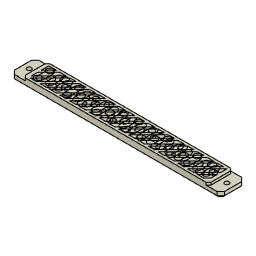
Front Panel - Master (Autodesk Fusion 360 design; units mm, degrees)
Autodesk Fusion 360 part; units mm, degrees
ref_plane "WorkPlane1" through (0, -117.8, 0) normal (0, 1, 0) x (0, 0, 1)
ref_plane "WorkPlane2" through (0, -123, 0) normal (0, 1, 0) x (0, 0, 1)
sketch "Master Sketch" plane through (0, -123, 0) normal (0, 1, 0) x (1, 0, 0)
  line L0 (-88.4862, 0.0071) -> (88.5, 0.0071) construction
  line L1 (88.5, 0.0071) -> (88.5, -28.9292)
  line L2 (88.5, -28.9292) -> (87.9405, -29.5447) construction
  line L3 (-88.4655, 0) -> (-88.4655, -26.8517) construction
  line L4 (-88.4862, -26.8517) -> (89.2, -26.8517) construction
  line L5 (89.2, -26.8517) -> (89.2, 0) construction
  line L6 (88.5, -26.8517) -> (88.5, 0.0071)
  line L7 (-88.4862, -26.8517) -> (88.5, -26.8517)
  line L8 (88.5, 0.0071) -> (-88.4862, 0.0071)
  line L9 (-88.4862, -26.8517) -> (-88.4862, 0.0071)
  line L10 (85.5, -21.8517) -> (85.5, -7.8517)
  line L11 (-82.4864, -24.8517) -> (82.5, -24.8517)
  line L12 (82.5, -4.8517) -> (-82.4864, -4.8517)
  line L13 (-88.4655, -4.8517) -> (-88.5, -4.8517)
  line L14 (-85.4864, -21.8517) -> (-85.4864, -7.8517)
  line L15 (-85.4864, 0.0071) -> (-85.4864, 0.0039)
  line L16 (-75.4864, -24.8517) -> (-75.4864, -4.8517)
  line L17 (75.5, -24.8517) -> (75.5, -4.8517)
  line L18 (-75.4864, -4.8517) -> (-80.4972, -4.8517)
  line L19 (-85.4864, -24.8517) -> (-75.4864, -24.8517) construction
  line L20 (-80.4864, -24.8517) -> (-80.4972, -4.8517) construction
  line L21 (0.0068, -24.8517) -> (0.0068, -4.8517) construction
  arc A0 (-82.4864, -4.8517) -> (-85.4864, -7.8517) centre (-82.4864, -7.8517) ccw construction
  arc A1 (-85.4864, -21.8517) -> (-82.4864, -24.8517) centre (-82.4864, -21.8517) ccw construction
  arc A2 (85.5, -7.8517) -> (82.5, -4.8517) centre (82.5, -7.8517) ccw construction
  arc A3 (82.5, -24.8517) -> (85.5, -21.8517) centre (82.5, -21.8517) ccw construction
  circle A4 centre (-80.4836, -14.7936) radius 1.8
  circle A5 centre (80.4971, -14.7936) radius 1.8
  line L22 (-85.4864, -21.8517) -> (-82.4864, -24.8517)
  line L23 (-85.4864, -7.8517) -> (-82.4864, -4.8517)
  line L24 (85.5, -7.8517) -> (82.5, -4.8517)
  line L25 (85.5, -21.8517) -> (82.4977, -24.8517)
  point P0 (85.5, -4.8517)
  point P1 (85.5, -24.8517)
  dimension "d919" = 2
  dimension "d922" = 20
  dimension "d925" = 10
  dimension "d926" = 10
  dimension "d928" = 3
  dimension "d929" = 3
  dimension "d930" = 3
  dimension "d931" = 3
  dimension "d932" = 3.6
  constraint coincident L4 L6.start
  constraint coincident L1 L6.start
  constraint coincident L0.end L1.start
  constraint coincident L4.start L7.start
  constraint coincident L0.start L8.end
  constraint parallel L7 L11
  constraint parallel L9 L14
  constraint parallel L8 L12
  constraint coincident L3 L13.start
  constraint collinear L12 L13
  constraint coincident L0 L15.start
  constraint collinear L14 L15
  constraint parallel L6 L10
  constraint parallel L10 L17
  constraint coincident L11 L17.start
  constraint coincident L12 L17.end
  constraint parallel L14 L16
  constraint perpendicular L14 L18
  constraint perpendicular L16 L19
  constraint midpoint L19 L20.start
  constraint coincident L12 L21.end
  constraint tangent L12 A0
  constraint tangent L14 A0
  constraint coincident L11 L21.start
  constraint coincident L19.start L14
  constraint coincident L11 L19.start
  constraint tangent L14 A1
  constraint tangent L11 A1
  constraint coincident L12 P0
  constraint coincident L10 P0
  constraint tangent L12 A2
  constraint tangent L10 A2
  constraint coincident L11 P1
  constraint coincident L10 P1
  constraint tangent L11 A3
  constraint tangent L10 A3
  constraint symmetric L21 A4 A5
  constraint coincident L12 L16.end
  constraint coincident L11 L16.start
  constraint vertical L16
  constraint horizontal L12
  constraint vertical L10
  constraint symmetric L21 L12.end L12.start
  constraint symmetric L21 L14.end L10.end
  constraint symmetric L21 L14.start L10.start
  constraint coincident L11 L25.end
  constraint coincident L10 A3.end
  constraint coincident L10 A2.start
  measures "d919" distance of L7 L11
  measures "d922" distance of P0 P1
  measures "d925" distance of L10 L17
  measures "d926" distance of L14 L16
  measures "d928" radius of A0
  measures "d929" radius of A1
  measures "d930" radius of A2
  measures "d931" radius of A3
  measures "d932" diameter of A4
extrude "Extrude1" add sketch "Master Sketch" along normal blind 4 contours L11 L12 L16 L17 makes body 1
extrude "Extrude2" add sketch "Master Sketch" along normal blind 2 contours L10 L11 L12 L17 L24 L25 | L11 L12 L14 L16 L18 L22 L23 bodies 1
chamfer "Chamfer1" distance 2 angle 45 4 edges at (-75.4864, -120, 24.8517) (-75.4864, -120, 4.8517) (75.5, -120, 4.8517) (75.5, -120, 24.8517) on bodies 1
move_body "Move1" bodies 1 to x (1, 0, 0) y (0, 0, 1) z (0, -1, 0) at (0, -118.1483, 127.8517)
extrude "Extrude3" add 3 faces at (-25.1576, -129.6667, 4.8517) (-79.352, -140.2322, 4.8517) (79.3648, -140.2322, 4.8517) along direction (0, 0, -1) blind 3 on bodies 1 bodies 1
chamfer "Chamfer2" distance 2 angle 45 8 edges at (85.5, -133, 1.8517) (83.9988, -141.5, 1.8517) (0.0056, -143, 1.8517) (-83.9864, -141.5, 1.8517) (-85.4864, -133, 1.8517) (-83.9864, -124.5, 1.8517) (0.0068, -123, 1.8517) (84, -124.5, 1.8517) on bodies 1
copy_body "Body->Comp1" bodies 1 removing the originals makes body 2 in component "Master"
sketch "Outline" plane through (0, -117.8, 0) normal (0, 1, 0) x (1, 0, 0) in component "Master"
  line L0 (-88.4655, -26.8517) -> (89.2, -26.8517)
  line L1 (89.2, -26.8517) -> (89.2, 0)
  line L2 (89.2, 0) -> (-88.4655, 0)
  line L3 (-88.4655, 0) -> (-88.4655, -26.8517)
sketch "USB A Panel Mount" plane through (0.0068, -133, 8.8517) normal (0, 0, 1) x (-1, 0, 0) in component "USB Sketches"
  line L0 (-73.4932, 10) -> (-75.4932, 8)
  line L1 (-75.4932, 8) -> (-75.4932, -8)
  line L2 (-75.4932, -8) -> (-73.4932, -10)
  line L3 (-73.4932, -10) -> (73.4932, -10)
  line L4 (73.4932, -10) -> (75.4932, -8)
  line L5 (75.4932, -8) -> (75.4932, 8)
  line L6 (75.4932, 8) -> (73.4932, 10)
  line L7 (73.4932, 10) -> (-73.4932, 10)
  line L8 (72.4932, 7.5) -> (33.4932, 7.5)
  line L9 (33.4932, 7.5) -> (33.4932, -7.5)
  line L10 (33.4932, -7.5) -> (72.4932, -7.5)
  line L11 (72.4932, -7.5) -> (72.4932, 7.5)
  line L12 (45.7432, -6) -> (60.2432, -6)
  line L13 (60.2432, -6) -> (60.2432, 6)
  line L14 (45.7432, 6) -> (45.7432, -6)
  line L15 (60.2432, 6) -> (45.7432, 6)
  circle A0 centre (68.2432, 0) radius 1.8
  circle A1 centre (37.7432, 0) radius 1.8
sketch "USB C Panel Mount" plane through (0.0068, -133, 8.8517) normal (0, 0, 1) x (-1, 0, 0) in component "USB Sketches"
  line L0 (-73.4932, 10) -> (-75.4932, 8)
  line L1 (-75.4932, 8) -> (-75.4932, -8)
  line L2 (-75.4932, -8) -> (-73.4932, -10)
  line L3 (-73.4932, -10) -> (73.4932, -10)
  line L4 (73.4932, -10) -> (75.4932, -8)
  line L5 (75.4932, -8) -> (75.4932, 8)
  line L6 (75.4932, 8) -> (73.4932, 10)
  line L7 (73.4932, 10) -> (-73.4932, 10)
  line L8 (72.4932, 6) -> (47.4932, 6)
  line L9 (47.4932, 6) -> (47.4932, -6)
  line L10 (47.4932, -6) -> (72.4932, -6)
  line L11 (72.4932, -6) -> (72.4932, 6)
  arc A0 (63.4932, -2.5) -> (64.4932, -1.5) centre (63.4932, -1.5) ccw
  line L12 (64.4932, 0) -> (64.4932, -1.5)
  line L13 (59.9932, -2.5) -> (63.4932, -2.5)
  arc A1 (55.4932, -1.5) -> (56.4932, -2.5) centre (56.4932, -1.5) ccw
  line L14 (55.4932, 0) -> (55.4932, -1.5)
  line L15 (59.9932, -2.5) -> (56.4932, -2.5)
  arc A2 (56.4932, 2.5) -> (55.4932, 1.5) centre (56.4932, 1.5) ccw
  line L16 (55.4932, 0) -> (55.4932, 1.5)
  line L17 (59.9932, 2.5) -> (56.4932, 2.5)
  circle A3 centre (51.6182, 0) radius 1.75
  circle A4 centre (68.3682, 0) radius 1.75
  arc A5 (64.4932, 1.5) -> (63.4932, 2.5) centre (63.4932, 1.5) ccw
  line L18 (59.9932, 2.5) -> (63.4932, 2.5)
  line L19 (64.4932, 0) -> (64.4932, 1.5)
sketch "Micro SD Slot" plane through (0, 0, 8.8517) normal (0, 0, 1) x (-1, 0, 0) in component "Master"
  line L0 (-73.5, 143) -> (-75.5, 141)
  line L1 (-75.5, 141) -> (-75.5, 125)
  line L2 (-75.5, 125) -> (-73.5, 123)
  line L3 (-73.5, 123) -> (73.4864, 123)
  line L4 (73.4864, 123) -> (75.4864, 125)
  line L5 (75.4864, 125) -> (75.4864, 141)
  line L6 (75.4864, 141) -> (73.4864, 143)
  line L7 (73.4864, 143) -> (-73.5, 143)
  line L8 (26.05, 129.6) -> (2.25, 129.6)
  line L9 (2.25, 129.6) -> (2.25, 136.4)
  line L10 (2.25, 136.4) -> (26.05, 136.4)
  line L11 (26.05, 136.4) -> (26.05, 129.6)
  line L12 (14.15, 132.9821) -> (28.75, 132.9821) construction
  line L13 (14.15, 132.9821) -> (14.15, 136.4) construction
  circle A0 centre (28.75, 132.9821) radius 1.8
  circle A1 centre (-0.45, 132.9821) radius 1.8
  line L14 (33.4864, 140.5) -> (33.4864, 125.5)
  line L15 (33.4864, 125.5) -> (-5.1864, 125.5)
  line L16 (-5.1864, 125.5) -> (-5.1864, 140.4642)
  line L17 (-5.1864, 140.4642) -> (33.4864, 140.4642)
  line L18 (33.4864, 140.4642) -> (33.4864, 125.5)
  line L19 (33.4864, 125.5) -> (-5.1864, 140.4642) construction
  line L20 (-5.1864, 125.5) -> (33.4864, 140.4642) construction
  line L21 (32.65, 129.5821) -> (-4.35, 129.5821)
  line L22 (-4.35, 129.5821) -> (-4.35, 136.3821)
  line L23 (-4.35, 136.3821) -> (32.65, 136.3821)
  line L24 (32.65, 136.3821) -> (32.65, 129.5821)
  line L25 (32.65, 129.5821) -> (-4.35, 136.3821) construction
  line L26 (-4.35, 129.5821) -> (32.65, 136.3821) construction
  point P0 (14.15, 132.9821)
  point P1 (14.15, 132.9821)
  point P2 (14.15, 132.9821)
  point P3 (14.15, 132.9821)
  dimension "d11" = 23.8
  dimension "d12" = 6.8
  dimension "d13" = 14.6
  dimension "d14" = 3.6
  dimension "d48" = 37
  dimension "d49" = 6.8
  constraint horizontal L8
  constraint perpendicular L8 L9
  constraint parallel L8 L10
  constraint parallel L9 L11
  constraint coincident P3 P2
  constraint perpendicular L11 L12
  constraint midpoint L10 L13.end
  constraint perpendicular L10 L13
  constraint coincident L12.end A0.centre
  constraint symmetric L13 A0 A1
  constraint horizontal L15
  constraint perpendicular L15 L16
  constraint parallel L15 L17
  constraint parallel L16 L18
  constraint coincident L19 P3
  constraint coincident L20 P3
  constraint coincident L14.end L15.start
  constraint horizontal L21
  constraint perpendicular L21 L22
  constraint parallel L21 L23
  constraint parallel L22 L24
  constraint coincident L25 P3
  constraint coincident L26 P3
  measures "d11" distance of L9.end L10.end
  measures "d12" distance of L8.end L9.end
  measures "d13" distance of P3 L12.end
  measures "d14" diameter of A0
  measures "d48" distance of L22.end L23.end
  measures "d49" distance of L21.end L22.end
sketch "Vent Sections" plane through (0, 0, 8.8517) normal (0, 0, 1) x (-1, 0, 0) in component "Vent Sketches"
  line L0 (-73.5, 143) -> (-75.5, 141)
  line L1 (-75.5, 141) -> (-75.5, 125)
  line L2 (-75.5, 125) -> (-73.5, 123)
  line L3 (-73.5, 123) -> (73.4864, 123)
  line L4 (73.4864, 123) -> (75.4864, 125)
  line L5 (75.4864, 125) -> (75.4864, 141)
  line L6 (75.4864, 141) -> (73.4864, 143)
  line L7 (73.4864, 143) -> (-73.5, 143)
  line L8 (33.4864, 140.4642) -> (33.4864, 125.5) construction
  line L9 (-5.1864, 125.5) -> (-5.1864, 140.4642) construction
  line L10 (-72.5, 141) -> (-72.5, 125)
  line L11 (72.4864, 125) -> (72.4864, 141)
  line L12 (72.4864, 141) -> (-72.5, 141)
  line L13 (-72.5, 125) -> (72.4864, 125)
  line L14 (-5.1864, 141) -> (-5.1864, 125)
  line L15 (33.4864, 141) -> (33.4864, 125)
  dimension "d15" = -3
  dimension "d17" = -3
  constraint perpendicular L10 L12
  constraint perpendicular L11 L13
  constraint coincident L12 L14.start
  constraint coincident L13 L14.end
  constraint perpendicular L13 L14
  constraint collinear L9 L14
  constraint coincident L12 L15.start
  constraint coincident L13 L15.end
  constraint perpendicular L13 L15
  constraint collinear L8 L15
sketch "Slots" plane through (0, 0, 8.8517) normal (0, 0, 1) x (-1, 0, 0) in component "Vent Sketches"
  line L0 (-73.5, 143) -> (-75.5, 141)
  line L1 (-75.5, 141) -> (-75.5, 125)
  line L2 (-75.5, 125) -> (-73.5, 123)
  line L3 (-73.5, 123) -> (73.4864, 123)
  line L4 (73.4864, 123) -> (75.4864, 125)
  line L5 (75.4864, 125) -> (75.4864, 141)
  line L6 (75.4864, 141) -> (73.4864, 143)
  line L7 (73.4864, 143) -> (-73.5, 143)
  line L8 (72.4864, 141) -> (-72.5, 141)
  line L9 (-72.5, 141) -> (-72.5, 125)
  line L10 (-72.5, 125) -> (72.4864, 125)
  line L11 (72.4864, 125) -> (72.4864, 141)
  line L12 (-5.1864, 141) -> (-5.1864, 125)
  line L13 (33.4864, 141) -> (33.4864, 125)
  line L14 (-0.0068, 141) -> (-0.0068, 125) construction
  line L15 (2.4932, 129) -> (2.4932, 137)
  arc A0 (2.4932, 137) -> (-2.5068, 137) centre (-0.0068, 137) ccw
  line L16 (-2.5068, 137) -> (-2.5068, 129)
  arc A1 (-2.5068, 129) -> (2.4932, 129) centre (-0.0068, 129) ccw
  line L17 (-0.0068, 129) -> (-0.0068, 137) construction
  line L18 (-70.0068, 137) -> (-70.0068, 129)
  arc A2 (-70.0068, 129) -> (-65.0068, 129) centre (-67.5068, 129) ccw
  line L19 (-65.0068, 129) -> (-65.0068, 137)
  arc A3 (-65.0068, 137) -> (-70.0068, 137) centre (-67.5068, 137) ccw
  line L20 (-62.5068, 137) -> (-62.5068, 129)
  arc A4 (-62.5068, 129) -> (-57.5068, 129) centre (-60.0068, 129) ccw
  line L21 (-57.5068, 129) -> (-57.5068, 137)
  arc A5 (-57.5068, 137) -> (-62.5068, 137) centre (-60.0068, 137) ccw
  line L22 (-55.0068, 137) -> (-55.0068, 129)
  arc A6 (-55.0068, 129) -> (-50.0068, 129) centre (-52.5068, 129) ccw
  line L23 (-50.0068, 129) -> (-50.0068, 137)
  arc A7 (-50.0068, 137) -> (-55.0068, 137) centre (-52.5068, 137) ccw
  line L24 (-47.5068, 137) -> (-47.5068, 129)
  arc A8 (-47.5068, 129) -> (-42.5068, 129) centre (-45.0068, 129) ccw
  line L25 (-42.5068, 129) -> (-42.5068, 137)
  arc A9 (-42.5068, 137) -> (-47.5068, 137) centre (-45.0068, 137) ccw
  line L26 (-40.0068, 137) -> (-40.0068, 129)
  arc A10 (-40.0068, 129) -> (-35.0068, 129) centre (-37.5068, 129) ccw
  line L27 (-35.0068, 129) -> (-35.0068, 137)
  arc A11 (-35.0068, 137) -> (-40.0068, 137) centre (-37.5068, 137) ccw
  line L28 (-32.5068, 137) -> (-32.5068, 129)
  arc A12 (-32.5068, 129) -> (-27.5068, 129) centre (-30.0068, 129) ccw
  line L29 (-27.5068, 129) -> (-27.5068, 137)
  arc A13 (-27.5068, 137) -> (-32.5068, 137) centre (-30.0068, 137) ccw
  line L30 (-25.0068, 137) -> (-25.0068, 129)
  arc A14 (-25.0068, 129) -> (-20.0068, 129) centre (-22.5068, 129) ccw
  line L31 (-20.0068, 129) -> (-20.0068, 137)
  arc A15 (-20.0068, 137) -> (-25.0068, 137) centre (-22.5068, 137) ccw
  line L32 (-17.5068, 137) -> (-17.5068, 129)
  arc A16 (-17.5068, 129) -> (-12.5068, 129) centre (-15.0068, 129) ccw
  line L33 (-12.5068, 129) -> (-12.5068, 137)
  arc A17 (-12.5068, 137) -> (-17.5068, 137) centre (-15.0068, 137) ccw
  line L34 (-10.0068, 137) -> (-10.0068, 129)
  arc A18 (-10.0068, 129) -> (-5.0068, 129) centre (-7.5068, 129) ccw
  line L35 (-5.0068, 129) -> (-5.0068, 137)
  arc A19 (-5.0068, 137) -> (-10.0068, 137) centre (-7.5068, 137) ccw
  line L36 (4.9932, 137) -> (4.9932, 129)
  arc A20 (4.9932, 129) -> (9.9932, 129) centre (7.4932, 129) ccw
  line L37 (9.9932, 129) -> (9.9932, 137)
  arc A21 (9.9932, 137) -> (4.9932, 137) centre (7.4932, 137) ccw
  line L38 (12.4932, 137) -> (12.4932, 129)
  arc A22 (12.4932, 129) -> (17.4932, 129) centre (14.9932, 129) ccw
  line L39 (17.4932, 129) -> (17.4932, 137)
  arc A23 (17.4932, 137) -> (12.4932, 137) centre (14.9932, 137) ccw
  line L40 (19.9932, 137) -> (19.9932, 129)
  arc A24 (19.9932, 129) -> (24.9932, 129) centre (22.4932, 129) ccw
  line L41 (24.9932, 129) -> (24.9932, 137)
  arc A25 (24.9932, 137) -> (19.9932, 137) centre (22.4932, 137) ccw
  line L42 (27.4932, 137) -> (27.4932, 129)
  arc A26 (27.4932, 129) -> (32.4932, 129) centre (29.9932, 129) ccw
  line L43 (32.4932, 129) -> (32.4932, 137)
  arc A27 (32.4932, 137) -> (27.4932, 137) centre (29.9932, 137) ccw
  line L44 (34.9932, 137) -> (34.9932, 129)
  arc A28 (34.9932, 129) -> (39.9932, 129) centre (37.4932, 129) ccw
  line L45 (39.9932, 129) -> (39.9932, 137)
  arc A29 (39.9932, 137) -> (34.9932, 137) centre (37.4932, 137) ccw
  line L46 (42.4932, 137) -> (42.4932, 129)
  arc A30 (42.4932, 129) -> (47.4932, 129) centre (44.9932, 129) ccw
  line L47 (47.4932, 129) -> (47.4932, 137)
  arc A31 (47.4932, 137) -> (42.4932, 137) centre (44.9932, 137) ccw
  line L48 (49.9932, 137) -> (49.9932, 129)
  arc A32 (49.9932, 129) -> (54.9932, 129) centre (52.4932, 129) ccw
  line L49 (54.9932, 129) -> (54.9932, 137)
  arc A33 (54.9932, 137) -> (49.9932, 137) centre (52.4932, 137) ccw
  line L50 (57.4932, 137) -> (57.4932, 129)
  arc A34 (57.4932, 129) -> (62.4932, 129) centre (59.9932, 129) ccw
  line L51 (62.4932, 129) -> (62.4932, 137)
  arc A35 (62.4932, 137) -> (57.4932, 137) centre (59.9932, 137) ccw
  line L52 (64.9932, 137) -> (64.9932, 129)
  arc A36 (64.9932, 129) -> (69.9932, 129) centre (67.4932, 129) ccw
  line L53 (69.9932, 129) -> (69.9932, 137)
  arc A37 (69.9932, 137) -> (64.9932, 137) centre (67.4932, 137) ccw
  point P0 (-0.0068, 133)
  dimension "d18" = 5
  dimension "d21" = 7.5
  dimension "d22" = 0
  constraint midpoint L8 L14.start
  constraint midpoint L10 L14.end
  constraint tangent L15 A0
  constraint tangent A0 L16
  constraint parallel L15 L16
  constraint tangent L16 A1
  constraint tangent L15 A1
  constraint perpendicular L8 L17
  constraint midpoint L14 P0
  constraint midpoint L17 P0
  measures "d18" diameter of A0
sketch "Slats" plane through (0, 0, 8.8517) normal (0, 0, 1) x (-1, 0, 0) in component "Vent Sketches"
  line L0 (-73.5, 143) -> (-75.5, 141)
  line L1 (-75.5, 141) -> (-75.5, 125)
  line L2 (-75.5, 125) -> (-73.5, 123)
  line L3 (-73.5, 123) -> (73.4864, 123)
  line L4 (73.4864, 123) -> (75.4864, 125)
  line L5 (75.4864, 125) -> (75.4864, 141)
  line L6 (75.4864, 141) -> (73.4864, 143)
  line L7 (73.4864, 143) -> (-73.5, 143)
  line L8 (72.4864, 141) -> (-72.5, 141)
  line L9 (-72.5, 141) -> (-72.5, 125)
  line L10 (72.4864, 125) -> (72.4864, 141)
  line L11 (-72.5, 125) -> (72.4864, 125)
  line L12 (-5.1864, 141) -> (-5.1864, 125)
  line L13 (33.4864, 141) -> (33.4864, 125)
  line L14 (-72.5, 125) -> (-56.4903, 141)
  line L15 (-69.5, 125) -> (-53.4903, 141)
  line L16 (-61.5, 125) -> (-45.4903, 141)
  line L17 (-64.5, 125) -> (-48.4903, 141)
  line L18 (-53.5, 125) -> (-37.4903, 141)
  line L19 (-56.5, 125) -> (-40.4903, 141)
  line L20 (-45.5, 125) -> (-29.4903, 141)
  line L21 (-48.5, 125) -> (-32.4903, 141)
  line L22 (-37.5, 125) -> (-21.4903, 141)
  line L23 (-40.5, 125) -> (-24.4903, 141)
  line L24 (-29.5, 125) -> (-13.4903, 141)
  line L25 (-32.5, 125) -> (-16.4903, 141)
  line L26 (-21.5, 125) -> (-5.4903, 141)
  line L27 (-24.5, 125) -> (-8.4903, 141)
  line L28 (-13.5, 125) -> (2.5097, 141)
  line L29 (-16.5, 125) -> (-0.4903, 141)
  line L30 (-5.5, 125) -> (10.5097, 141)
  line L31 (-8.5, 125) -> (7.5097, 141)
  line L32 (2.5, 125) -> (18.5097, 141)
  line L33 (-0.5, 125) -> (15.5097, 141)
  line L34 (10.5, 125) -> (26.5097, 141)
  line L35 (7.5, 125) -> (23.5097, 141)
  line L36 (18.5, 125) -> (34.5097, 141)
  line L37 (15.5, 125) -> (31.5097, 141)
  line L38 (26.5, 125) -> (42.5097, 141)
  line L39 (23.5, 125) -> (39.5097, 141)
  line L40 (34.5, 125) -> (50.5097, 141)
  line L41 (31.5, 125) -> (47.5097, 141)
  line L42 (42.5, 125) -> (58.5097, 141)
  line L43 (39.5, 125) -> (55.5097, 141)
  line L44 (50.5, 125) -> (66.5097, 141)
  line L45 (47.5, 125) -> (63.5097, 141)
  line L46 (58.5, 125) -> (74.5097, 141)
  line L47 (55.5, 125) -> (71.5097, 141)
  line L48 (66.5, 125) -> (82.5097, 141)
  line L49 (63.5, 125) -> (79.5097, 141)
  line L50 (-72.5, 137.9921) -> (-69.4903, 141)
  line L51 (-72.5, 140.9903) -> (-72.4903, 141)
  line L52 (-72.5, 132.9951) -> (-64.4903, 141)
  line L53 (-72.5, 129.997) -> (-61.4903, 141)
  dimension "d25" = 8
  dimension "d26" = 0
  constraint coincident L9.end L11.start
  constraint coincident L8 L14.end
  constraint coincident L8 L15.end
  constraint coincident L11 L15.start
  constraint parallel L14 L15
  constraint coincident L9 L50.start
  constraint coincident L9 L51.start
  constraint coincident L9 L52.start
  constraint coincident L9 L53.start
sketch "Hexagons" plane through (0, 0, 8.8517) normal (0, 0, 1) x (-1, 0, 0) in component "Vent Sketches"
  line L0 (-73.5, 143) -> (-75.5, 141)
  line L1 (-75.5, 141) -> (-75.5, 125)
  line L2 (-75.5, 125) -> (-73.5, 123)
  line L3 (-73.5, 123) -> (73.4864, 123)
  line L4 (73.4864, 123) -> (75.4864, 125)
  line L5 (75.4864, 125) -> (75.4864, 141)
  line L6 (75.4864, 141) -> (73.4864, 143)
  line L7 (73.4864, 143) -> (-73.5, 143)
  line L8 (-72.5, 125) -> (72.4864, 125)
  line L9 (72.4864, 125) -> (72.4864, 141)
  line L10 (-72.5, 141) -> (-72.5, 125)
  line L11 (72.4864, 141) -> (-72.5, 141)
  line L12 (-5.1864, 141) -> (-5.1864, 125)
  line L13 (33.4864, 141) -> (33.4864, 125)
  line L14 (-72.5, 133) -> (-69.5, 133) construction
  line L15 (-66.5, 133) -> (-68, 135.5981)
  line L16 (-68, 135.5981) -> (-71, 135.5981)
  line L17 (-71, 135.5981) -> (-72.5, 133)
  line L18 (-72.5, 133) -> (-71, 130.4019)
  line L19 (-71, 130.4019) -> (-68, 130.4019)
  line L20 (-68, 130.4019) -> (-66.5, 133)
  line L21 (-65, 140.5981) -> (-66.5, 138)
  line L22 (-66.5, 138) -> (-65, 135.4019)
  line L23 (-65, 135.4019) -> (-62, 135.4019)
  line L24 (-62, 135.4019) -> (-60.5, 138)
  line L25 (-60.5, 138) -> (-62, 140.5981)
  line L26 (-62, 140.5981) -> (-65, 140.5981)
  line L27 (-62, 125.4019) -> (-65, 125.4019)
  line L28 (-65, 125.4019) -> (-66.5, 128)
  line L29 (-66.5, 128) -> (-65, 130.5981)
  line L30 (-65, 130.5981) -> (-62, 130.5981)
  line L31 (-62, 130.5981) -> (-60.5, 128)
  line L32 (-60.5, 128) -> (-62, 125.4019)
  line L33 (-50, 125.4019) -> (-53, 125.4019)
  line L34 (-53, 125.4019) -> (-54.5, 128)
  line L35 (-54.5, 128) -> (-53, 130.5981)
  line L36 (-53, 130.5981) -> (-50, 130.5981)
  line L37 (-50, 130.5981) -> (-48.5, 128)
  line L38 (-48.5, 128) -> (-50, 125.4019)
  line L39 (-56, 135.5981) -> (-59, 135.5981)
  line L40 (-59, 135.5981) -> (-60.5, 133)
  line L41 (-60.5, 133) -> (-59, 130.4019)
  line L42 (-59, 130.4019) -> (-56, 130.4019)
  line L43 (-54.5, 133) -> (-56, 135.5981)
  line L44 (-56, 130.4019) -> (-54.5, 133)
  line L45 (-48.5, 138) -> (-50, 140.5981)
  line L46 (-50, 140.5981) -> (-53, 140.5981)
  line L47 (-53, 140.5981) -> (-54.5, 138)
  line L48 (-54.5, 138) -> (-53, 135.4019)
  line L49 (-50, 135.4019) -> (-48.5, 138)
  line L50 (-53, 135.4019) -> (-50, 135.4019)
  line L51 (-38, 125.4019) -> (-41, 125.4019)
  line L52 (-41, 125.4019) -> (-42.5, 128)
  line L53 (-42.5, 128) -> (-41, 130.5981)
  line L54 (-41, 130.5981) -> (-38, 130.5981)
  line L55 (-38, 130.5981) -> (-36.5, 128)
  line L56 (-36.5, 128) -> (-38, 125.4019)
  line L57 (-44, 135.5981) -> (-47, 135.5981)
  line L58 (-47, 135.5981) -> (-48.5, 133)
  line L59 (-48.5, 133) -> (-47, 130.4019)
  line L60 (-47, 130.4019) -> (-44, 130.4019)
  line L61 (-42.5, 133) -> (-44, 135.5981)
  line L62 (-44, 130.4019) -> (-42.5, 133)
  line L63 (-36.5, 138) -> (-38, 140.5981)
  line L64 (-38, 140.5981) -> (-41, 140.5981)
  line L65 (-41, 140.5981) -> (-42.5, 138)
  line L66 (-42.5, 138) -> (-41, 135.4019)
  line L67 (-38, 135.4019) -> (-36.5, 138)
  line L68 (-41, 135.4019) -> (-38, 135.4019)
  line L69 (-26, 125.4019) -> (-29, 125.4019)
  line L70 (-29, 125.4019) -> (-30.5, 128)
  line L71 (-30.5, 128) -> (-29, 130.5981)
  line L72 (-29, 130.5981) -> (-26, 130.5981)
  line L73 (-26, 130.5981) -> (-24.5, 128)
  line L74 (-24.5, 128) -> (-26, 125.4019)
  line L75 (-32, 135.5981) -> (-35, 135.5981)
  line L76 (-35, 135.5981) -> (-36.5, 133)
  line L77 (-36.5, 133) -> (-35, 130.4019)
  line L78 (-35, 130.4019) -> (-32, 130.4019)
  line L79 (-30.5, 133) -> (-32, 135.5981)
  line L80 (-32, 130.4019) -> (-30.5, 133)
  line L81 (-24.5, 138) -> (-26, 140.5981)
  line L82 (-26, 140.5981) -> (-29, 140.5981)
  line L83 (-29, 140.5981) -> (-30.5, 138)
  line L84 (-30.5, 138) -> (-29, 135.4019)
  line L85 (-26, 135.4019) -> (-24.5, 138)
  line L86 (-29, 135.4019) -> (-26, 135.4019)
  line L87 (-14, 125.4019) -> (-17, 125.4019)
  line L88 (-17, 125.4019) -> (-18.5, 128)
  line L89 (-18.5, 128) -> (-17, 130.5981)
  line L90 (-17, 130.5981) -> (-14, 130.5981)
  line L91 (-14, 130.5981) -> (-12.5, 128)
  line L92 (-12.5, 128) -> (-14, 125.4019)
  line L93 (-20, 135.5981) -> (-23, 135.5981)
  line L94 (-23, 135.5981) -> (-24.5, 133)
  line L95 (-24.5, 133) -> (-23, 130.4019)
  line L96 (-23, 130.4019) -> (-20, 130.4019)
  line L97 (-18.5, 133) -> (-20, 135.5981)
  line L98 (-20, 130.4019) -> (-18.5, 133)
  line L99 (-12.5, 138) -> (-14, 140.5981)
  line L100 (-14, 140.5981) -> (-17, 140.5981)
  line L101 (-17, 140.5981) -> (-18.5, 138)
  line L102 (-18.5, 138) -> (-17, 135.4019)
  line L103 (-14, 135.4019) -> (-12.5, 138)
  line L104 (-17, 135.4019) -> (-14, 135.4019)
  line L105 (-2, 125.4019) -> (-5, 125.4019)
  line L106 (-5, 125.4019) -> (-6.5, 128)
  line L107 (-6.5, 128) -> (-5, 130.5981)
  line L108 (-5, 130.5981) -> (-2, 130.5981)
  line L109 (-2, 130.5981) -> (-0.5, 128)
  line L110 (-0.5, 128) -> (-2, 125.4019)
  line L111 (-8, 135.5981) -> (-11, 135.5981)
  line L112 (-11, 135.5981) -> (-12.5, 133)
  line L113 (-12.5, 133) -> (-11, 130.4019)
  line L114 (-11, 130.4019) -> (-8, 130.4019)
  line L115 (-6.5, 133) -> (-8, 135.5981)
  line L116 (-8, 130.4019) -> (-6.5, 133)
  line L117 (-0.5, 138) -> (-2, 140.5981)
  line L118 (-2, 140.5981) -> (-5, 140.5981)
  line L119 (-5, 140.5981) -> (-6.5, 138)
  line L120 (-6.5, 138) -> (-5, 135.4019)
  line L121 (-2, 135.4019) -> (-0.5, 138)
  line L122 (-5, 135.4019) -> (-2, 135.4019)
  line L123 (10, 125.4019) -> (7, 125.4019)
  line L124 (7, 125.4019) -> (5.5, 128)
  line L125 (5.5, 128) -> (7, 130.5981)
  line L126 (7, 130.5981) -> (10, 130.5981)
  line L127 (10, 130.5981) -> (11.5, 128)
  line L128 (11.5, 128) -> (10, 125.4019)
  line L129 (4, 135.5981) -> (1, 135.5981)
  line L130 (1, 135.5981) -> (-0.5, 133)
  line L131 (-0.5, 133) -> (1, 130.4019)
  line L132 (1, 130.4019) -> (4, 130.4019)
  line L133 (5.5, 133) -> (4, 135.5981)
  line L134 (4, 130.4019) -> (5.5, 133)
  line L135 (11.5, 138) -> (10, 140.5981)
  line L136 (10, 140.5981) -> (7, 140.5981)
  line L137 (7, 140.5981) -> (5.5, 138)
  line L138 (5.5, 138) -> (7, 135.4019)
  line L139 (10, 135.4019) -> (11.5, 138)
  line L140 (7, 135.4019) -> (10, 135.4019)
  line L141 (22, 125.4019) -> (19, 125.4019)
  line L142 (19, 125.4019) -> (17.5, 128)
  line L143 (17.5, 128) -> (19, 130.5981)
  line L144 (19, 130.5981) -> (22, 130.5981)
  line L145 (22, 130.5981) -> (23.5, 128)
  line L146 (23.5, 128) -> (22, 125.4019)
  line L147 (16, 135.5981) -> (13, 135.5981)
  line L148 (13, 135.5981) -> (11.5, 133)
  line L149 (11.5, 133) -> (13, 130.4019)
  line L150 (13, 130.4019) -> (16, 130.4019)
  line L151 (17.5, 133) -> (16, 135.5981)
  line L152 (16, 130.4019) -> (17.5, 133)
  line L153 (23.5, 138) -> (22, 140.5981)
  line L154 (22, 140.5981) -> (19, 140.5981)
  line L155 (19, 140.5981) -> (17.5, 138)
  line L156 (17.5, 138) -> (19, 135.4019)
  line L157 (22, 135.4019) -> (23.5, 138)
  line L158 (19, 135.4019) -> (22, 135.4019)
  line L159 (34, 125.4019) -> (31, 125.4019)
  line L160 (31, 125.4019) -> (29.5, 128)
  line L161 (29.5, 128) -> (31, 130.5981)
  line L162 (31, 130.5981) -> (34, 130.5981)
  line L163 (34, 130.5981) -> (35.5, 128)
  line L164 (35.5, 128) -> (34, 125.4019)
  line L165 (28, 135.5981) -> (25, 135.5981)
  line L166 (25, 135.5981) -> (23.5, 133)
  line L167 (23.5, 133) -> (25, 130.4019)
  line L168 (25, 130.4019) -> (28, 130.4019)
  line L169 (29.5, 133) -> (28, 135.5981)
  line L170 (28, 130.4019) -> (29.5, 133)
  line L171 (35.5, 138) -> (34, 140.5981)
  line L172 (34, 140.5981) -> (31, 140.5981)
  line L173 (31, 140.5981) -> (29.5, 138)
  line L174 (29.5, 138) -> (31, 135.4019)
  line L175 (34, 135.4019) -> (35.5, 138)
  line L176 (31, 135.4019) -> (34, 135.4019)
  line L177 (46, 125.4019) -> (43, 125.4019)
  line L178 (43, 125.4019) -> (41.5, 128)
  line L179 (41.5, 128) -> (43, 130.5981)
  line L180 (43, 130.5981) -> (46, 130.5981)
  line L181 (46, 130.5981) -> (47.5, 128)
  line L182 (47.5, 128) -> (46, 125.4019)
  line L183 (40, 135.5981) -> (37, 135.5981)
  line L184 (37, 135.5981) -> (35.5, 133)
  line L185 (35.5, 133) -> (37, 130.4019)
  line L186 (37, 130.4019) -> (40, 130.4019)
  line L187 (41.5, 133) -> (40, 135.5981)
  line L188 (40, 130.4019) -> (41.5, 133)
  line L189 (47.5, 138) -> (46, 140.5981)
  line L190 (46, 140.5981) -> (43, 140.5981)
  line L191 (43, 140.5981) -> (41.5, 138)
  line L192 (41.5, 138) -> (43, 135.4019)
  line L193 (46, 135.4019) -> (47.5, 138)
  line L194 (43, 135.4019) -> (46, 135.4019)
  line L195 (58, 125.4019) -> (55, 125.4019)
  line L196 (55, 125.4019) -> (53.5, 128)
  line L197 (53.5, 128) -> (55, 130.5981)
  line L198 (55, 130.5981) -> (58, 130.5981)
  line L199 (58, 130.5981) -> (59.5, 128)
  line L200 (59.5, 128) -> (58, 125.4019)
  line L201 (52, 135.5981) -> (49, 135.5981)
  line L202 (49, 135.5981) -> (47.5, 133)
  line L203 (47.5, 133) -> (49, 130.4019)
  line L204 (49, 130.4019) -> (52, 130.4019)
  line L205 (53.5, 133) -> (52, 135.5981)
  line L206 (52, 130.4019) -> (53.5, 133)
  line L207 (59.5, 138) -> (58, 140.5981)
  line L208 (58, 140.5981) -> (55, 140.5981)
  line L209 (55, 140.5981) -> (53.5, 138)
  line L210 (53.5, 138) -> (55, 135.4019)
  line L211 (58, 135.4019) -> (59.5, 138)
  line L212 (55, 135.4019) -> (58, 135.4019)
  line L213 (70, 125.4019) -> (67, 125.4019)
  line L214 (67, 125.4019) -> (65.5, 128)
  line L215 (65.5, 128) -> (67, 130.5981)
  line L216 (67, 130.5981) -> (70, 130.5981)
  line L217 (70, 130.5981) -> (71.5, 128)
  line L218 (71.5, 128) -> (70, 125.4019)
  line L219 (64, 135.5981) -> (61, 135.5981)
  line L220 (61, 135.5981) -> (59.5, 133)
  line L221 (59.5, 133) -> (61, 130.4019)
  line L222 (61, 130.4019) -> (64, 130.4019)
  line L223 (65.5, 133) -> (64, 135.5981)
  line L224 (64, 130.4019) -> (65.5, 133)
  line L225 (71.5, 138) -> (70, 140.5981)
  line L226 (70, 140.5981) -> (67, 140.5981)
  line L227 (67, 140.5981) -> (65.5, 138)
  line L228 (65.5, 138) -> (67, 135.4019)
  line L229 (70, 135.4019) -> (71.5, 138)
  line L230 (67, 135.4019) -> (70, 135.4019)
  point P0 (-69.5, 133)
  dimension "d31" = 3
  dimension "d32" = 3
  dimension "d35" = 12
  dimension "d36" = 0
  constraint midpoint L10 L14.start
  constraint perpendicular L10 L14
  constraint coincident P0 L14.end
  constraint symmetric L14 L21.end L28.end
  constraint symmetric L14 L23.end L30.end
  constraint symmetric L14 L24.end L31.end
  constraint symmetric L14 L25.end L27.start
  constraint symmetric L14 L21.start L27.end
  constraint symmetric L14 L22.end L29.end
  measures "d31" distance of L15.start P0
  measures "d32" distance of L14.start P0
copy_body "CopyPasteBodies1" bodies 2 makes body 3 in component "Master"
move_body "Move1'" bodies 3 to x (1, 0, 0) y (0, 1, 0) z (0, 0, 1) at (0, 0, 0) in component "Master"
extrude "Extrude1'" cut sketch "Hexagons" against normal blind 7 contours L15 L16 L17 L18 L19 L20 | L21 L22 L23 L24 L25 L26 | L27 L28 L29 L30 L31 L32 | L33 L34 L35 L36 L37 L38 | L39 L40 L41 L42 L43 L44 | L45 L46 L47 L48 L49 L50 | L51 L52 L53 L54 L55 L56 | L57 L58 L59 L60 L61 L62 | L63 L64 L65 L66 L67 L68 | L69 L70 L71 L72 L73 L74 | L75 L76 L77 L78 L79 L80 | L81 L82 L83 L84 L85 L86 | L87 L88 L89 L90 L91 L92 | L93 L94 L95 L96 L97 L98 | L99 L100 L101 L102 L103 L104 | L111 L112 L113 L114 L115 L116 bodies 3 in component "Master"
copy_body "CopyPasteBodies2" bodies 2 makes body 4 in component "Master"
move_body "Move2" bodies 4 to x (1, 0, 0) y (0, 1, 0) z (0, 0, 1) at (0, 0, 0) in component "Master"
extrude "Extrude2'" cut sketch "Slots" against normal through all contours L12 A18 L35 A19 | L12 L34 A18 A19 | L18 A2 L19 A3 | L20 A4 L21 A5 | L22 A6 L23 A7 | L24 A8 L25 A9 | L26 A10 L27 A11 | L28 A12 L29 A13 | L30 A14 L31 A15 | L32 A16 L33 A17 bodies 4 in component "Master"
copy_body "CopyPasteBodies3" bodies 2 makes body 5 in component "Master"
move_body "Move3" bodies 5 to x (1, 0, 0) y (0, 1, 0) z (0, 0, 1) at (0, 0, 0) in component "Master"
extrude "Extrude3'" cut sketch "Slats" against normal through all contours L11 L12 L28 L31 | L8 L11 L12 L26 L29 | L8 L11 L24 L27 | L8 L11 L22 L25 | L8 L11 L20 L23 | L8 L11 L18 L21 | L8 L11 L16 L19 | L8 L11 L15 L17 | L8 L9 L14 L53 | L8 L9 L50 L52 bodies 5 in component "Master"
copy_body "CopyPasteBodies1'" bodies 4 makes body 6 in component "Vent Only Slots"
move_body "Move1''" bodies 6 to x (1, 0, 0) y (0, 1, 0) z (0, 0, 1) at (0, 0, 0) in component "Vent Only Slots"
extrude "Extrude1''" cut sketch "Slots" against normal through all contours L15 A0 L16 A1 | L36 A20 L37 A21 | L38 A22 L39 A23 | L40 A24 L41 A25 | L42 A26 L43 A27 | L44 A28 L45 A29 | L46 A30 L47 A31 | L48 A32 L49 A33 | L50 A34 L51 A35 | L52 A36 L53 A37 bodies 6 in component "Vent Only Slots"
copy_body "CopyPasteBodies1''" bodies 5 makes body 7 in component "Vent Only Slats"
move_body "Move1'''" bodies 7 to x (1, 0, 0) y (0, 1, 0) z (0, 0, 1) at (0, 0, 0) in component "Vent Only Slats"
extrude "Extrude1'''" cut sketch "Slats" against normal through all contours L10 L11 L46 L49 | L10 L11 L48 | L8 L11 L44 L47 | L8 L11 L42 L45 | L8 L11 L40 L43 | L8 L13 L38 L41 | L11 L13 L38 L41 | L8 L13 L36 L39 | L11 L13 L36 L39 | L8 L11 L34 L37 | L8 L11 L32 L35 | L8 L11 L12 L30 L33 | L8 L12 L28 L31 | L8 L12 L29 bodies 7 in component "Vent Only Slats"
copy_body "CopyPasteBodies1'''" bodies 3 makes body 8 in component "Vent Only Hexagons"
move_body "Move1''''" bodies 8 to x (1, 0, 0) y (0, 1, 0) z (0, 0, 1) at (0, 0, 0) in component "Vent Only Hexagons"
extrude "Extrude1''''" cut sketch "Hexagons" against normal through all contours L12 L106 L107 | L12 L105 L106 L107 L108 L109 L110 | L13 L159 L160 L161 L162 | L13 L159 L162 L163 L164 | L12 L119 L120 | L12 L117 L118 L119 L120 L121 L122 | L13 L172 L173 L174 L176 | L13 L171 L172 L175 L176 | L123 L124 L125 L126 L127 L128 | L129 L130 L131 L132 L133 L134 | L135 L136 L137 L138 L139 L140 | L141 L142 L143 L144 L145 L146 | L147 L148 L149 L150 L151 L152 | L153 L154 L155 L156 L157 L158 | L165 L166 L167 L168 L169 L170 | L177 L178 L179 L180 L181 L182 | L183 L184 L185 L186 L187 L188 | L189 L190 L191 L192 L193 L194 | L195 L196 L197 L198 L199 L200 | L201 L202 L203 L204 L205 L206 | L207 L208 L209 L210 L211 L212 | L213 L214 L215 L216 L217 L218 | L219 L220 L221 L222 L223 L224 | L225 L226 L227 L228 L229 L230 bodies 8 in component "Vent Only Hexagons"
copy_body "CopyPasteBodies1''''" bodies 3 4 5 makes body 9 makes body 10 makes body 11 in component "No USB"
move_body "Move1'''''" bodies 9 10 11 to x (1, 0, 0) y (0, 1, 0) z (0, 0, 1) at (0, 0, 0) in component "No USB"
extrude "Extrude1'''''" cut sketch "Micro SD Slot" against normal blind 7 contours L8 L9 L11 L23 | L9 L10 L11 L23 | A0 | A1 bodies 9 10 11 in component "No USB"
extrude "Extrude2''" cut sketch "Micro SD Slot" against normal blind 5 contours L8 L9 L11 L21 L22 L23 L24 bodies 9 10 11 in component "No USB"
copy_body "CopyPasteBodies2'" bodies 9 10 11 makes body 12 makes body 13 makes body 14 in component "USB C"
move_body "Move2'" bodies 12 13 14 to x (1, 0, 0) y (0, 1, 0) z (0, 0, 1) at (0, 0, 0) in component "USB C"
copy_body "CopyPasteBodies1'''''" bodies 9 10 11 makes body 15 makes body 16 makes body 17 in component "USB A"
move_body "Move1''''''" bodies 15 16 17 to x (1, 0, 0) y (0, 1, 0) z (0, 0, 1) at (0, 0, 0) in component "USB A"
extrude "Extrude3''" cut sketch "Hexagons" against normal blind 8 contours L177 L178 L179 L180 L181 L182 | L183 L184 L185 L186 L187 L188 | L189 L190 L191 L192 L193 L194 | L195 L196 L197 L198 L199 L200 | L201 L202 L203 L204 L205 L206 | L207 L208 L209 L210 L211 L212 | L213 L214 L215 L216 L217 L218 | L219 L220 L221 L222 L223 L224 | L225 L226 L227 L228 L229 L230 bodies 9 in component "No USB"
copy_body "Body->Comp1'" bodies 9 removing the originals makes body 18 in component "MicroSD, Hexagons"
extrude "Extrude4" cut sketch "Slots" against normal blind 8 contours L44 A28 L45 A29 | L46 A30 L47 A31 | L48 A32 L49 A33 | L50 A34 L51 A35 | L52 A36 L53 A37 bodies 10 in component "No USB"
copy_body "CutPasteBodies1" bodies 10 removing the originals makes body 19 in component "MicroSD, Slots"
extrude "Extrude5" cut sketch "Slats" against normal blind 8 contours L10 L11 L46 L49 | L10 L11 L48 | L8 L11 L44 L47 | L8 L11 L42 L45 | L8 L11 L40 L43 | L8 L13 L38 L41 | L8 L13 L36 L39 bodies 11 in component "No USB"
copy_body "Body->Comp2" bodies 11 removing the originals makes body 20 in component "MicroSD, Slats"
extrude "Extrude1''''''" cut sketch "USB A Panel Mount" against normal blind 7 contours L12 L13 L14 L15 | A0 | A1 bodies 15 16 17 in component "USB A"
extrude "Extrude2'''" cut sketch "USB A Panel Mount" against normal blind 4 contours L8 L9 L10 L11 bodies 15 16 17 in component "USB A"
copy_body "Body->Comp1''" bodies 15 removing the originals makes body 21 in component "MicroSD, USB A, Hexagons"
copy_body "Body->Comp2'" bodies 17 removing the originals makes body 22 in component "MicroSD, USB A, Slats"
copy_body "Body->Comp3" bodies 16 removing the originals makes body 23 in component "MicroSD, USB A, Slots"
extrude "Extrude1'''''''" cut sketch "USB C Panel Mount" against normal blind 7 contours A0 L12 L13 A1 L14 L15 A2 L16 L17 A5 L18 L19 | A3 | A4 bodies 12 13 14 in component "USB C"
extrude "Extrude2''''" cut sketch "USB C Panel Mount" against normal blind 4 contours L8 L9 L10 L11 bodies 12 13 14 in component "USB C"
copy_body "Body->Comp1'''" bodies 12 removing the originals makes body 24 in component "MicroSD, USB C, Hexagons"
copy_body "Body->Comp2''" bodies 13 removing the originals makes body 25 in component "MicroSD, USB C, Slots"
copy_body "Body->Comp3'" bodies 14 removing the originals makes body 26 in component "MicroSD, USB C, Slats"
component "Master" placed x (1, 0, 0) y (0, 1, 0) z (0, 0, 1) at (0, 0, 0)
component "USB C" placed x (1, 0, 0) y (0, 1, 0) z (0, 0, 1) at (0, 0, 0)
component "USB A" placed x (1, 0, 0) y (0, 1, 0) z (0, 0, 1) at (0, 0, 0)
component "No USB" placed x (1, 0, 0) y (0, 1, 0) z (0, 0, 1) at (0, 0, 0)
component "Vent Only" placed x (1, 0, 0) y (0, 1, 0) z (0, 0, 1) at (0, 0, 0)
component "USB Sketches" placed x (1, 0, 0) y (0, 1, 0) z (0, 0, 1) at (0, 0, 0) in component "Master"
component "Vent Sketches" placed x (1, 0, 0) y (0, 1, 0) z (0, 0, 1) at (0, 0, 0) in component "Master"
component "MicroSD, USB C, Hexagons" placed x (1, 0, 0) y (0, 1, 0) z (0, 0, 1) at (0, 0, 0) in component "USB C"
component "MicroSD, USB C, Slots" placed x (1, 0, 0) y (0, 1, 0) z (0, 0, 1) at (0, 0, 0) in component "USB C"
component "MicroSD, USB C, Slats" placed x (1, 0, 0) y (0, 1, 0) z (0, 0, 1) at (0, 0, 0) in component "USB C"
component "MicroSD, USB A, Hexagons" placed x (1, 0, 0) y (0, 1, 0) z (0, 0, 1) at (0, 0, 0) in component "USB A"
component "MicroSD, USB A, Slats" placed x (1, 0, 0) y (0, 1, 0) z (0, 0, 1) at (0, 0, 0) in component "USB A"
component "MicroSD, USB A, Slots" placed x (1, 0, 0) y (0, 1, 0) z (0, 0, 1) at (0, 0, 0) in component "USB A"
component "MicroSD, Slots" placed x (1, 0, 0) y (0, 1, 0) z (0, 0, 1) at (0, 0, 0) in component "No USB"
component "MicroSD, Hexagons" placed x (1, 0, 0) y (0, 1, 0) z (0, 0, 1) at (0, 0, 0) in component "No USB"
component "MicroSD, Slats" placed x (1, 0, 0) y (0, 1, 0) z (0, 0, 1) at (0, 0, 0) in component "No USB"
component "Vent Only Slots" placed x (1, 0, 0) y (0, 1, 0) z (0, 0, 1) at (0, 0, 0) in component "Vent Only"
component "Vent Only Slats" placed x (1, 0, 0) y (0, 1, 0) z (0, 0, 1) at (0, 0, 0) in component "Vent Only"
component "Vent Only Hexagons" placed x (1, 0, 0) y (0, 1, 0) z (0, 0, 1) at (0, 0, 0) in component "Vent Only"
hidden bodies 2 3 4 5
equation "d932 = large_m3"
equation "large_m3 = 3.6 mm"
equation "d13 = ( 29.2 / 2 ) * 1 mm"
named bodies: "Blank", "Hexagons", "Slots", "Slats"
